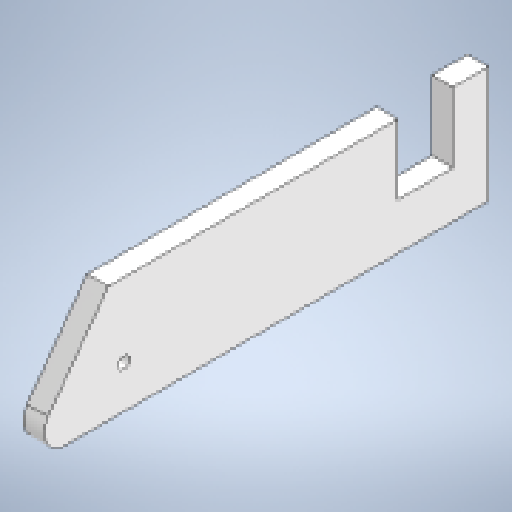
# Autodesk Inventor part: Side
Saved by Autodesk Inventor 2023.2 (Build 272271000, 271)
## iProperties
Created: 2023-11-13
Part Number: Side
Material: UHMW, White
Document SubType Name: Modeling
Designer: Nathan Cai
Density: 0.94 g/cm^3
Appearance: Smooth - White
Mass: 24.2041 g
Surface Area: 104.152 cm^2
Volume: 25.749 cm^3
Author: Nathan Cai
Autodesk Inventor part; units mm, degrees
ref_plane "YZ Plane" through (0, 0, 0) normal (1, 0, 0) x (0, 1, 0)
ref_plane "XZ Plane" through (0, 0, 0) normal (0, 1, 0) x (-1, 0, 0)
ref_plane "XY Plane" through (0, 0, 0) normal (0, 0, 1) x (1, 0, 0)
sketch "Sketch1" plane through (0, 0, 0) normal (1, 0, 0) x (0, 1, 0)
  line L0 (-17.4625, 57.15) -> (17.4625, 57.15)
  line L1 (17.4625, 57.15) -> (17.4625, -57.15)
  line L2 (17.4625, -57.15) -> (-17.4625, -57.15)
  line L3 (-17.4625, -57.15) -> (-17.4625, 57.15)
  line L4 (-17.4625, 57.15) -> (17.4625, -57.15) construction
  line L5 (17.4625, 57.15) -> (-17.4625, -57.15) construction
  line L6 (0, 57.15) -> (0, -57.15) construction
  circle A0 centre (4.7625, -38.1) radius 12.7 construction
  line L7 (17.4625, -50.8) -> (-17.4625, -50.8) construction
  circle A1 centre (4.7625, -38.1) radius 11
  line L8 (-17.4625, 57.15) -> (17.4625, 57.15)
  line L9 (17.4625, 57.15) -> (17.4625, 82.55) construction
  line L10 (17.4625, 82.55) -> (-17.4625, 82.55) construction
  line L11 (-17.4625, 82.55) -> (-17.4625, 57.15)
  line L12 (-17.4625, 82.55) -> (17.4625, 57.15)
  circle A2 centre (4.7625, -38.1) radius 25.4 construction
  line L13 (17.4625, -25.4) -> (-17.4625, -25.4) construction
  line L14 (-3.4875, -46.35) -> (13.0125, -46.35)
  line L15 (13.0125, -46.35) -> (13.0125, -29.85) construction
  line L16 (13.0125, -29.85) -> (-3.4875, -29.85)
  line L17 (-3.4875, -29.85) -> (-3.4875, -46.35)
  line L18 (-3.4875, -46.35) -> (13.0125, -29.85) construction
  line L19 (13.0125, -46.35) -> (-3.4875, -29.85) construction
  line L20 (-3.4875, -46.35) -> (17.4625, -46.35)
  line L21 (17.4625, -46.35) -> (17.4625, -29.85)
  line L22 (17.4625, -29.85) -> (-3.4875, -29.85)
  line L23 (-3.4875, -29.85) -> (-3.4875, -46.35)
  circle A3 centre (-4.7625, 52.3875) radius 15.875
  line L24 (-20.6375, -38.1) -> (-20.6375, 52.3875) construction
  circle A4 centre (-4.7625, 52.3875) radius 1.7526
  point P0 (0, 0)
  point P1 (14.2875, -46.35)
  point P2 (14.2875, -29.85)
  point P3 (12.0383, -29.85)
  point P4 (17.4625, -32.5978)
  point P5 (17.4625, -43.6022)
  point P6 (12.0383, -46.35)
  point P7 (17.4625, -46.35)
  dimension "d9" = 50.8
  dimension "d16" = 31.75
  dimension "d0" = 34.925
  dimension "d1" = 114.3
  dimension "d2" = 25.4
  dimension "d6" = 22
  dimension "d7" = 25.4
  dimension "d11" = 6.35
  dimension "d12" = 16.5
  dimension "d13" = 16.5
  dimension "d15" = 12.7
  dimension "d17" = 90.4875
  dimension "d18" = 3.5052
  constraints: 50 end point, 8 parallel, 7 point on line, 6 midpoint, 6 perpendicular, 4 horizontal, 3 centre point, 3 coincident, 3 vertical, 2 horizontal alignment, 2 tangent, 4 other
  measures "d0" distance of L1.end L2.end
  measures "d1" distance of L0.end L1.end
  measures "d2" diameter of A0
  measures "d6" diameter of A1
  measures "d7" distance of L9.end L8.end
  measures "d11" distance between parallel lines of L2 L7
  measures "d12" distance of L16.end L15.end
  measures "d13" distance of L15.end L14.end
  measures "d15" distance from line of L1 A1.centre
  measures "d17" vertical distance of point (-4.762, 52.388) point (4.763, -38.1)
  measures "d18" diameter of A4
extrude "Extrusion1" add sketch "Sketch1" along normal blind 6.35 contours L11 A3 L0 | L0 A3 L3 | A3 L11 L12 L0 | L0 L1 L22 L16 A1 L17 L14 L20 L2 L3 A3 | L16 A1 | A1 L14 | L17 A1
fillet "Fillet1" radius 6.35 1 edges at (3.175, -17.4625, 82.55)
body "Solid1"
